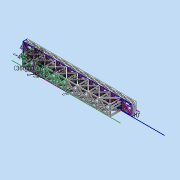
# Autodesk Inventor part: hashi1shado
Saved by Autodesk Inventor 2022 (Build 260153000, 153)
## iProperties
Created: 2024-05-14
Part Number: hashi1shado
Material: 一般
Document SubType Name: Modeling
Designer: ktamu
Density: 1 g/cm^3
Appearance: 既定
Mass: 212.611 g
Surface Area: 1968.28 cm^2
Volume: 212.611 cm^3
Author: ktamu
Autodesk Inventor part; units mm, degrees
(part 1 of 2)
ref_plane "YZ Plane" through (0, 0, 0) normal (1, 0, 0) x (0, 1, 0)
ref_plane "XZ Plane" through (0, 0, 0) normal (0, 1, 0) x (-1, 0, 0)
ref_plane "XY Plane" through (0, 0, 0) normal (0, 0, 1) x (1, 0, 0)
sketch "スケッチ2" plane through (0, 0, 0) normal (1, 0, 0) x (0, 1, 0)
  line L0 (25, 10) -> (-25, 10)
  line L1 (-25, 10) -> (-25, -10)
  line L2 (-25, -10) -> (25, -10)
  line L3 (25, -10) -> (25, 10)
  line L4 (25, 10) -> (-25, -10) construction
  line L5 (-25, 10) -> (25, -10) construction
  point P0 (0, 0)
  dimension "d4" = 50
  dimension "d5" = 20
  constraints: 12 end point, 2 midpoint, 2 parallel, 1 horizontal, 1 perpendicular
  measures "d4" distance of L2.end L1.end
  measures "d5" distance of L1.end L0.end
extrude "押し出し2" add sketch "スケッチ2" along normal mid plane 500
sketch "スケッチ3" plane through (-250, -25, 10) normal (0, 0, 1) x (1, 0, 0)
  circle A0 centre (250, 25) radius 5
  dimension "d8" = 10
  constraints: 1 centre point, 1 coincident
  measures "d8" diameter of A0
extrude "押し出し3" add sketch "スケッチ3" along normal blind 2
sketch "SCfront" plane through (-250, -25, 10) normal (0, -1, 0) x (1, 0, 0)
  line L0 (0, -20) -> (500, -20) projected
  line L1 (500, 0) -> (500, -20) projected
  line L2 (500, 0) -> (0, 0) projected
  line L3 (0, -20) -> (0, 0) projected
  line L4 (0, 0) -> (500, 0)
  line L5 (500, 0) -> (500, -20)
  line L6 (500, -20) -> (0, -20)
  line L7 (0, -20) -> (0, 0)
  line L8 (0, 0) -> (500, -20) construction
  line L9 (500, 0) -> (0, -20) construction
  line L10 (0, 0) -> (500, 0) projected
  line L11 (0, -20) -> (500, -20) projected
  line L12 (0, 0) -> (50, 0)
  line L13 (50, 0) -> (50, -20)
  line L14 (50, -20) -> (0, -20)
  line L15 (0, -20) -> (0, 0)
  line L16 (100, 0) -> (100, -20)
  line L17 (150, 0) -> (150, -20)
  line L18 (200, 0) -> (200, -20)
  line L19 (250, 0) -> (250, -20)
  line L20 (450, 0) -> (450, -20)
  line L21 (400, 0) -> (400, -20)
  line L22 (350, 0) -> (350, -20)
  line L23 (300, 0) -> (300, -20)
  line L24 (0, 0) -> (0, -20) projected
  line L25 (0, 0) -> (50, -20)
  line L26 (0, -20) -> (50, 0) construction
  line L27 (50, 0) -> (100, -20)
  line L28 (100, 0) -> (50, -20)
  line L29 (52, -4) -> (98, -4)
  line L30 (98, -4) -> (98, -16)
  line L31 (98, -16) -> (52, -16)
  line L32 (52, -16) -> (52, -4)
  line L33 (75, -10) -> (98, -16) construction
  line L34 (98, -4) -> (52, -16) construction
  line L35 (102, -4) -> (148, -4)
  line L36 (102, -16) -> (102, -4)
  line L37 (148, -16) -> (102, -16)
  line L38 (148, -4) -> (148, -16)
  line L39 (152, -4) -> (198, -4)
  line L40 (152, -16) -> (152, -4)
  line L41 (198, -16) -> (152, -16)
  line L42 (198, -4) -> (198, -16)
  line L43 (202, -4) -> (248, -4)
  line L44 (202, -16) -> (202, -4)
  line L45 (248, -16) -> (202, -16)
  line L46 (248, -4) -> (248, -16)
  line L47 (252, -4) -> (298, -4)
  line L48 (252, -16) -> (252, -4)
  line L49 (298, -16) -> (252, -16)
  line L50 (298, -4) -> (298, -16)
  line L51 (302, -4) -> (348, -4)
  line L52 (302, -16) -> (302, -4)
  line L53 (348, -16) -> (302, -16)
  line L54 (348, -4) -> (348, -16)
  line L55 (352, -4) -> (398, -4)
  line L56 (352, -16) -> (352, -4)
  line L57 (398, -16) -> (352, -16)
  line L58 (398, -4) -> (398, -16)
  line L59 (402, -4) -> (448, -4)
  line L60 (402, -16) -> (402, -4)
  line L61 (448, -16) -> (402, -16)
  line L62 (448, -4) -> (448, -16)
  line L63 (48, -4) -> (48, -16)
  line L64 (48, -4) -> (4, -4)
  line L65 (4, -4) -> (4, -16.3421)
  line L66 (4, -16.3421) -> (48, -16.3421)
  line L67 (48, -16.3421) -> (48, -4)
  line L68 (452, -4) -> (452, -16)
  line L69 (452, -4) -> (496, -4)
  line L70 (496, -4) -> (496, -16.3421)
  line L71 (496, -16.3421) -> (452, -16.3421)
  line L72 (11.4052, -4) -> (48, -14.2649)
  line L73 (4, -6.0772) -> (40.5948, -16.3421)
  line L74 (488.5948, -4) -> (452, -14.2649)
  line L75 (496, -6.0772) -> (459.4052, -16.3421)
  line L76 (52, -4) -> (75, -10)
  line L77 (52, -6.0669) -> (90.0768, -16)
  line L78 (52.5048, -2.0648) -> (52.6652, -2.1066)
  line L79 (59.9232, -4) -> (98, -13.9331)
  line L80 (109.9232, -4) -> (148, -13.9331)
  line L81 (102, -6.0669) -> (140.0768, -16)
  line L82 (159.9232, -4) -> (198, -13.9331)
  line L83 (152, -6.0669) -> (190.0768, -16)
  line L84 (209.9232, -4) -> (248, -13.9331)
  line L85 (202, -6.0669) -> (240.0768, -16)
  line L86 (448, -6.0669) -> (409.9232, -16)
  line L87 (440.0768, -4) -> (402, -13.9331)
  line L88 (390.0768, -4) -> (352, -13.9331)
  line L89 (398, -6.0669) -> (359.9232, -16)
  line L90 (340.0768, -4) -> (302, -13.9331)
  line L91 (348, -6.0669) -> (309.9232, -16)
  line L92 (290.0768, -4) -> (252, -13.9331)
  line L93 (298, -6.0669) -> (259.9232, -16)
  line L94 (0, -10) -> (496, -10) construction
  line L95 (0, -10) -> (496, -10) construction
  line L96 (11.4052, -16) -> (48, -5.7351)
  line L97 (4, -13.9228) -> (39.375, -4)
  line L98 (488.5948, -16) -> (452, -5.7351)
  line L99 (496, -13.9228) -> (459.4052, -3.6579)
  line L100 (52, -13.9331) -> (90.0768, -4)
  line L101 (59.9232, -16) -> (98, -6.0669)
  line L102 (109.9232, -16) -> (148, -6.0669)
  line L103 (102, -13.9331) -> (140.0768, -4)
  line L104 (159.9232, -16) -> (198, -6.0669)
  line L105 (152, -13.9331) -> (190.0768, -4)
  line L106 (209.9232, -16) -> (248, -6.0669)
  line L107 (202, -13.9331) -> (240.0768, -4)
  line L108 (448, -13.9331) -> (409.9232, -4)
  line L109 (440.0768, -16) -> (402, -6.0669)
  line L110 (398, -13.9331) -> (359.9232, -4)
  line L111 (390.0768, -16) -> (352, -6.0669)
  line L112 (348, -13.9331) -> (309.9232, -4)
  line L113 (340.0768, -16) -> (302, -6.0669)
  line L114 (298, -13.9331) -> (259.9232, -4)
  line L115 (290.0768, -16) -> (252, -6.0669)
  line L116 (25.3901, -12.0772) -> (10.1855, -16.3421)
  line L117 (474.6099, -12.0772) -> (489.8145, -16.3421)
  line L118 (50.8793, -20) -> (54.8793, -20)
  line L119 (54.8793, -20) -> (54.8793, -36)
  line L120 (54.8793, -36) -> (50.8793, -36)
  line L121 (50.8793, -36) -> (50.8793, -20)
  line L122 (500, -20) -> (0, -20)
  line L123 (0, -36) -> (500, -36)
  line L124 (445.1207, -20) -> (445.1207, -36)
  line L125 (449.1207, -36) -> (449.1207, -20)
  line L126 (50, 0) -> (100, 0)
  line L127 (100, 0) -> (100, 50)
  line L128 (100, 50) -> (50, 50)
  line L129 (50, 50) -> (50, 0)
  line L130 (50, 50) -> (100, 0)
  line L131 (50, 0) -> (100, 50)
  line L132 (50, 0) -> (100, 0)
  line L133 (54.8284, 48) -> (95.1716, 48)
  line L134 (95.1716, 48) -> (75, 27.8284)
  line L135 (75, 27.8284) -> (54.8284, 48)
  line L136 (52, 4.8284) -> (52, 45.1716)
  line L137 (72.1716, 25) -> (52, 4.8284)
  line L138 (52, 45.1716) -> (72.1716, 25)
  line L139 (95.1716, 2) -> (54.8284, 2)
  line L140 (75, 22.1716) -> (95.1716, 2)
  line L141 (54.8284, 2) -> (75, 22.1716)
  line L142 (98, 45.1716) -> (98, 4.8284)
  line L143 (77.8284, 25) -> (98, 45.1716)
  line L144 (98, 4.8284) -> (77.8284, 25)
  line L145 (55.944, 3.1156) -> (52.8284, 0)
  line L146 (93.8909, 3.2807) -> (97.1716, 0)
  line L147 (150, 50) -> (100, 50)
  line L148 (104.8284, 48) -> (145.1716, 48)
  line L149 (145.1716, 48) -> (125, 27.8284)
  line L150 (125, 27.8284) -> (104.8284, 48)
  line L151 (102, 4.8284) -> (102, 45.1716)
  line L152 (102, 45.1716) -> (122.1716, 25)
  line L153 (122.1716, 25) -> (102, 4.8284)
  line L154 (127.8284, 25) -> (148, 45.1716)
  line L155 (148, 45.1716) -> (148, 4.8284)
  line L156 (148, 4.8284) -> (127.8284, 25)
  line L157 (104.8284, 2) -> (125, 22.1716)
  line L158 (125, 22.1716) -> (145.1716, 2)
  line L159 (143.8909, 3.2807) -> (147.1716, 0)
  line L160 (50, 0) -> (550, 0)
  line L161 (105.944, 3.1156) -> (102.8284, 0)
  line L162 (200, 50) -> (150, 50)
  line L163 (154.8284, 48) -> (195.1716, 48)
  line L164 (195.1716, 48) -> (175, 27.8284)
  line L165 (175, 27.8284) -> (154.8284, 48)
  line L166 (152, 4.8284) -> (152, 45.1716)
  line L167 (152, 45.1716) -> (172.1716, 25)
  line L168 (172.1716, 25) -> (152, 4.8284)
  line L169 (177.8284, 25) -> (198, 45.1716)
  line L170 (198, 45.1716) -> (198, 4.8284)
  line L171 (198, 4.8284) -> (177.8284, 25)
  line L172 (154.8284, 2) -> (175, 22.1716)
  line L173 (175, 22.1716) -> (195.1716, 2)
  line L174 (193.8909, 3.2807) -> (197.1716, 0)
  line L175 (100, 0) -> (600, 0)
  line L176 (155.944, 3.1156) -> (152.8284, 0)
  line L177 (250, 50) -> (200, 50)
  line L178 (204.8284, 48) -> (245.1716, 48)
  line L179 (245.1716, 48) -> (225, 27.8284)
  line L180 (225, 27.8284) -> (204.8284, 48)
  line L181 (202, 4.8284) -> (202, 45.1716)
  line L182 (202, 45.1716) -> (222.1716, 25)
  line L183 (222.1716, 25) -> (202, 4.8284)
  line L184 (227.8284, 25) -> (248, 45.1716)
  line L185 (248, 45.1716) -> (248, 4.8284)
  line L186 (248, 4.8284) -> (227.8284, 25)
  line L187 (204.8284, 2) -> (225, 22.1716)
  line L188 (225, 22.1716) -> (245.1716, 2)
  line L189 (243.8909, 3.2807) -> (247.1716, 0)
  line L190 (150, 0) -> (650, 0)
  line L191 (205.944, 3.1156) -> (202.8284, 0)
  line L192 (250, 50) -> (250, 0)
  line L193 (250, 50) -> (250, 52)
  line L194 (250, 52) -> (50, 52)
  line L195 (50, 52) -> (50, 50)
  point P0 (250, -10)
  point P1 (440.0768, -4)
  point P2 (390.0768, -4)
  point P3 (340.0768, -4)
  point P4 (290.0768, -4)
  point P5 (209.9232, -4)
  point P6 (159.9232, -4)
  point P7 (109.9232, -4)
  point P8 (60.1439, -4.0576)
  point P9 (60, -4)
  point P10 (90, -16)
  point P11 (89.8561, -15.9424)
  point P12 (48, -14.2649)
  point P13 (40.5948, -3.6579)
  point P14 (482.0151, -10)
  point P15 (474.6099, -7.9228)
  point P16 (460.625, -4)
  point P17 (467.2046, -10)
  point P18 (432.9232, -10)
  point P19 (425, -12.0669)
  point P20 (425, -7.9331)
  point P21 (417.0768, -10)
  point P22 (382.9232, -10)
  point P23 (375, -12.0669)
  point P24 (375, -7.9331)
  point P25 (367.0768, -10)
  point P26 (332.9232, -10)
  point P27 (325, -12.0669)
  point P28 (325, -7.9331)
  point P29 (317.0768, -10)
  point P30 (282.9232, -10)
  point P31 (275, -12.0669)
  point P32 (275, -7.9331)
  point P33 (267.0768, -10)
  point P34 (232.9232, -10)
  point P35 (225, -7.9331)
  point P36 (225, -12.0669)
  point P37 (217.0768, -10)
  point P38 (182.9232, -10)
  point P39 (175, -7.9331)
  point P40 (175, -12.0669)
  point P41 (167.0768, -10)
  point P42 (132.9232, -10)
  point P43 (125, -7.9331)
  point P44 (125, -12.0669)
  point P45 (117.0768, -10)
  point P46 (67.0768, -10)
  point P47 (59.9232, -16)
  point P48 (75, -12.0669)
  point P49 (75, -7.9331)
  point P50 (82.9232, -10)
  point P51 (25.3901, -7.9228)
  point P52 (32.7954, -10)
  point P53 (48, -5.7351)
  point P54 (11.4052, -16)
  point P55 (17.9849, -10)
  point P56 (4, -13.9228)
  point P57 (54.8793, -20)
  point P58 (75, 25)
  point P59 (202.8284, 0)
  point P60 (152.8284, 0)
  point P61 (102.8284, 0)
  point P62 (54.8284, 2)
  point P63 (52.8284, 0)
  dimension "d12" = 50
  dimension "d15" = 50
  dimension "d20" = 46
  dimension "d21" = 12
  dimension "d24" = 50
  dimension "d29" = 4
  dimension "d30" = 4
  dimension "d33" = 4
  dimension "d37" = 2
  dimension "d40" = 50
  dimension "d96" = 0
  dimension "d97" = 10
  dimension "d116" = 4
  dimension "d125" = 50
  dimension "d126" = 50
  dimension "d132" = 2
  dimension "d133" = 2
  dimension "d134" = 2
  dimension "d137" = 360
  dimension "d141" = 50
  dimension "d146" = 2
  constraints: 378 end point, 79 symmetric about line, 41 point on line, 18 parallel, 12 horizontal, 7 midpoint, 6 perpendicular, 3 collinear, 1 vertical, 215 other
  measures "d12" distance of L13.end L14.end
  measures "d15" distance of L12.end L16.start
  measures "d20" distance of L30.end L31.end
  measures "d21" distance of L29.end L30.end
  measures "d24" distance of L29.start L35.start
  measures "d29" distance between parallel lines of L32 L63
  measures "d30" distance between parallel lines of L65 L3
  measures "d33" distance between parallel lines of L12 L64
  measures "d37" distance between parallel lines of L76 L77
  measures "d40" distance of L79.start L80.start
  measures "d96" distance between parallel lines of L94 L95
  measures "d97" distance between parallel lines of L0 L95
  measures "d116" distance of L119.end L120.end
  measures "d125" distance of L128.end L127.end
  measures "d126" distance of L127.end L126.end
  measures "d132" distance between parallel lines of L130 L135
  measures "d133" distance between parallel lines of L128 L133
  measures "d134" distance between parallel lines of L131 L134
  measures "d141" distance of L127.end L147.start
  measures "d146" distance of L193.end L193.start
extrude "押し出し4" cut sketch "SCfront" against normal through all contours L31 L101 L28 | L28 L101 L77 L27 L31 | L29 L28 L100 L79 L27 | L66 L116 L96 L73 | L101 L31 L32 L100 L77 L28 | L28 L77 L101 | L64 L97 L72 | L29 L100 L28 | L96 L116 L66 L65 L97 L73 | L96 L63 L72 | L72 L97 L64 L63 L96 | L97 L65 L73 | L100 L28 L79 | L100 L29 L30 L101 L79 L28 | L100 L32 L77 | L101 L30 L79 | L35 L103 L80 | L81 L103 L36 | L35 L38 L102 L80 L103 | L103 L81 L102 L37 L36 | L102 L38 L80 | L81 L37 L102 | L39 L105 L82 | L83 L105 L40 | L39 L42 L104 L82 L105 | L105 L83 L104 L41 L40 | L104 L42 L82 | L83 L41 L104 | L43 L107 L84 | L85 L107 L44 | L43 L46 L106 L84 L107 | L107 L85 L106 L45 L44 | L106 L46 L84 | L85 L45 L106 | L47 L114 L92 L115 L48 | L47 L92 L114 | L115 L92 L48 | L114 L50 L49 L115 L93 | L93 L50 L114 | L115 L49 L93 | L51 L112 L90 L113 L52 | L51 L90 L112 | L113 L90 L52 | L112 L54 L53 L113 L91 | L91 L54 L112 | L113 L53 L91 | L55 L110 L88 L111 L56 | L55 L88 L110 | L111 L88 L56 | L110 L58 L57 L111 L89 | L89 L58 L110 | L111 L57 L89 | L59 L108 L87 L109 L60 | L59 L87 L108 | L109 L87 L60 | L108 L62 L61 L109 L86 | L86 L62 L108 | L109 L61 L86 | L69 L99 L74 L98 L68 | L98 L74 L68 | L69 L74 L99 | L98 L117 L71 L75 | L75 L99 L70 L71 L117 L98 | L75 L70 L99
sketch "SCLeft" plane through (-250, 0, 0) normal (-1, 0, 0) x (0, 0, 1)
  line L0 (10, 25) -> (10, -25) projected
  line L1 (-10, 25) -> (10, 25)
  line L2 (10, 25) -> (10, -25)
  line L3 (10, -25) -> (-10, -25)
  line L4 (-10, -25) -> (-10, 25)
  line L5 (-10, 25) -> (10, -25) construction
  line L6 (10, 25) -> (-10, -25) construction
  line L7 (-6, 21) -> (6, 21)
  line L8 (6, 21) -> (6, -21)
  line L9 (6, -21) -> (-6, -21)
  line L10 (-6, -21) -> (-6, 21)
  line L11 (-6, 21) -> (-1.04, 3.6401) construction
  line L12 (6, 21) -> (-6, -21) construction
  line L13 (7.4154, 0) -> (4.3427, 0)
  line L14 (2.08, 0) -> (6, -13.7199)
  line L15 (-3.92, 21) -> (0, 7.2801)
  line L16 (-6, 21) -> (-1.04, 3.6401)
  line L17 (1.04, -3.6401) -> (6, -21)
  line L18 (-6, 13.7199) -> (-2.08, 0)
  line L19 (0, -7.2801) -> (3.92, -21)
  line L20 (0, 7.2801) -> (3.92, 21)
  line L21 (-6, -13.7199) -> (-2.08, 0)
  line L22 (-3.92, -21) -> (0, -7.2801)
  line L23 (2.08, 0) -> (6, 13.7199)
  point P0 (0, 0)
  dimension "d47" = 12
  dimension "d48" = 42
  constraints: 46 end point, 8 parallel, 5 point on line, 4 symmetric about line, 3 horizontal, 3 midpoint, 2 perpendicular
  measures "d47" distance of L8.end L9.end
  measures "d48" distance of L7.end L8.end
extrude "押し出し5left" cut sketch "SCLeft" against normal through all contours L7 L15 L20 L8 L23 L14 L9 L19 L22 L10 L21 L18 | L7 L20 L15 | L18 L21 L10 | L8 L14 L23 | L22 L19 L9
extrude "押し出し6" add sketch "SCLeft" against normal blind 4 contours L7 L15 L20 L8 L23 L14 L9 L19 L22 L10 L21 L18
mirror "ミラー1" about plane through (0, 0, 0) normal (1, 0, 0) of "押し出し6"
sketch "SCtop" plane through (-250, -25, 10) normal (0, 0, 1) x (1, 0, 0)
  circle A0 centre (250, 25) radius 5 projected
  line L0 (500, 0) -> (0, 0) projected
  line L1 (500, 50) -> (500, 0) projected
  line L2 (0, 50) -> (500, 50) projected
  line L3 (0, 0) -> (0, 50) projected
  circle A1 centre (250, 25) radius 5 projected
  line L4 (0, 0) -> (0, 50) projected
  line L5 (0, 50) -> (500, 0) construction
  line L6 (0, 0) -> (500, 0) projected
  line L7 (500, 50) -> (0, 0) construction
  line L8 (0, 50) -> (500, 50)
  line L9 (500, 50) -> (500, 0)
  line L10 (500, 0) -> (0, 0)
  line L11 (0, 0) -> (0, 50)
  line L12 (0, 50) -> (500, 0) construction
  line L13 (500, 50) -> (0, 0) construction
  line L14 (0, 50) -> (500, 50) projected
  line L15 (0, 50) -> (50, 50)
  line L16 (50, 50) -> (50, 0)
  line L17 (50, 0) -> (0, 0)
  line L18 (0, 0) -> (0, 50)
  line L19 (100, 50) -> (100, 0)
  line L20 (150, 50) -> (150, 0)
  line L21 (200, 50) -> (200, 0)
  line L22 (250, 50) -> (250, 0)
  line L23 (300, 50) -> (300, 0)
  line L24 (350, 50) -> (350, 0)
  line L25 (400, 50) -> (400, 0)
  line L26 (450, 50) -> (450, 0)
  line L27 (50, 50) -> (100, 0)
  line L28 (0, 50) -> (50, 0)
  line L29 (50, 50) -> (0, 0)
  line L30 (98, 4) -> (60.1439, 4) projected
  line L31 (52, 46) -> (98, 46)
  line L32 (98, 46) -> (98, 4)
  line L33 (98, 4) -> (52, 4)
  line L34 (52, 4) -> (52, 46)
  line L35 (4, 46) -> (48, 46)
  line L36 (48, 46) -> (48, 4)
  line L37 (48, 4) -> (4, 4)
  line L38 (4, 4) -> (4, 46)
  line L39 (6.8284, 46) -> (48.0258, 4.8026)
  line L40 (4, 43.1716) -> (43.1716, 4)
  line L41 (25, 25) -> (25, 18.6219)
  line L42 (98, 0) -> (98, 4) projected
  line L43 (53.4759, 44.6524) -> (98, 4)
  line L44 (52, 43.2918) -> (95.0338, 4)
  line L45 (54.9662, 46) -> (98, 6.7082)
  line L46 (98, 43.2918) -> (54.9662, 4)
  line L47 (92.2747, 40.7725) -> (53.4759, 5.3476)
  line L48 (95.0338, 46) -> (52, 6.7082)
  line L49 (50.1449, 5.0145) -> (50, 4.8822)
  line L50 (73.5843, 23.5843) -> (90.9091, 40.9091)
  line L51 (92.2747, 40.7725) -> (73.5169, 23.6459) construction
  line L52 (53.4759, 5.3476) -> (52, 4) construction
  line L53 (52, 46) -> (53.4759, 44.6524) construction
  line L54 (73.5169, 26.3541) -> (98, 4) construction
  line L55 (48, 46) -> (4, 4)
  line L56 (45.1034, 46) -> (4, 6.7649)
  line L57 (48, 43.2351) -> (6.8966, 4)
  line L58 (104.9662, 46) -> (148, 6.7082)
  line L59 (145.0338, 46) -> (102, 6.7082)
  line L60 (148, 43.2918) -> (104.9662, 4)
  line L61 (102, 43.2918) -> (145.0338, 4)
  line L62 (148, 46) -> (148, 4)
  line L63 (102, 46) -> (148, 46)
  line L64 (102, 4) -> (102, 46)
  line L65 (148, 4) -> (102, 4)
  line L66 (154.9662, 46) -> (198, 6.7082)
  line L67 (195.0338, 46) -> (152, 6.7082)
  line L68 (198, 43.2918) -> (154.9662, 4)
  line L69 (152, 43.2918) -> (195.0338, 4)
  line L70 (198, 46) -> (198, 4)
  line L71 (152, 46) -> (198, 46)
  line L72 (152, 4) -> (152, 46)
  line L73 (198, 4) -> (152, 4)
  line L74 (204.9662, 46) -> (248, 6.7082)
  line L75 (245.0338, 46) -> (202, 6.7082)
  line L76 (248, 43.2918) -> (204.9662, 4)
  line L77 (202, 43.2918) -> (245.0338, 4)
  line L78 (248, 46) -> (248, 4)
  line L79 (202, 46) -> (248, 46)
  line L80 (202, 4) -> (202, 46)
  line L81 (248, 4) -> (202, 4)
  line L82 (254.9662, 46) -> (298, 6.7082)
  line L83 (295.0338, 46) -> (252, 6.7082)
  line L84 (298, 43.2918) -> (254.9662, 4)
  line L85 (252, 43.2918) -> (295.0338, 4)
  line L86 (298, 46) -> (298, 4)
  line L87 (252, 46) -> (298, 46)
  line L88 (252, 4) -> (252, 46)
  line L89 (298, 4) -> (252, 4)
  line L90 (304.9662, 46) -> (348, 6.7082)
  line L91 (345.0338, 46) -> (302, 6.7082)
  line L92 (348, 43.2918) -> (304.9662, 4)
  line L93 (302, 43.2918) -> (345.0338, 4)
  line L94 (348, 46) -> (348, 4)
  line L95 (302, 46) -> (348, 46)
  line L96 (302, 4) -> (302, 46)
  line L97 (348, 4) -> (302, 4)
  line L98 (354.9662, 46) -> (398, 6.7082)
  line L99 (395.0338, 46) -> (352, 6.7082)
  line L100 (398, 43.2918) -> (354.9662, 4)
  line L101 (352, 43.2918) -> (395.0338, 4)
  line L102 (398, 46) -> (398, 4)
  line L103 (352, 46) -> (398, 46)
  line L104 (352, 4) -> (352, 46)
  line L105 (398, 4) -> (352, 4)
  line L106 (404.9662, 46) -> (448, 6.7082)
  line L107 (445.0338, 46) -> (402, 6.7082)
  line L108 (448, 43.2918) -> (404.9662, 4)
  line L109 (402, 43.2918) -> (445.0338, 4)
  line L110 (448, 46) -> (448, 4)
  line L111 (402, 46) -> (448, 46)
  line L112 (402, 4) -> (402, 46)
  line L113 (448, 4) -> (402, 4)
  line L114 (496, 46) -> (452, 46)
  line L115 (452, 46) -> (452, 4)
  line L116 (452, 4) -> (496, 4)
  line L117 (496, 4) -> (496, 46)
  line L118 (493.1716, 46) -> (451.9742, 4.8026)
  line L119 (496, 43.1716) -> (456.8284, 4)
  line L120 (454.8966, 46) -> (496, 6.7649)
  line L121 (452, 43.2351) -> (493.1034, 4)
  point P0 (75, 25)
  point P1 (123.5169, 26.3541)
  point P2 (123.5843, 23.5843)
  point P3 (123.5169, 23.6459)
  point P4 (173.5169, 26.3541)
  point P5 (173.5843, 23.5843)
  point P6 (173.5169, 23.6459)
  point P7 (223.5169, 26.3541)
  point P8 (223.5843, 23.5843)
  point P9 (223.5169, 23.6459)
  point P10 (273.5169, 26.3541)
  point P11 (273.5843, 23.5843)
  point P12 (273.5169, 23.6459)
  point P13 (323.5169, 26.3541)
  point P14 (323.5843, 23.5843)
  point P15 (323.5169, 23.6459)
  point P16 (373.5169, 26.3541)
  point P17 (373.5843, 23.5843)
  point P18 (373.5169, 23.6459)
  point P19 (423.5169, 26.3541)
  point P20 (423.5843, 23.5843)
  point P21 (423.5169, 23.6459)
  point P22 (474.5441, 21.7157)
  point P23 (477.3733, 24.5449)
  point P24 (474.4791, 27.3075)
  point P25 (452, 4.8284)
  point P26 (471.6499, 24.4784)
  point P27 (427.9662, 25)
  point P28 (425, 22.2918)
  point P29 (425, 27.7082)
  point P30 (375, 22.2918)
  point P31 (375, 27.7082)
  point P32 (422.0338, 25)
  point P33 (377.9662, 25)
  point P34 (372.0338, 25)
  point P35 (327.9662, 25)
  point P36 (325, 22.2918)
  point P37 (325, 27.7082)
  point P38 (322.0338, 25)
  point P39 (275, 22.2918)
  point P40 (277.9662, 25)
  point P41 (275, 27.7082)
  point P42 (252, 20.4174)
  point P43 (272.0338, 25)
  point P44 (252, 29.5826)
  point P45 (225, 22.2918)
  point P46 (248, 29.5826)
  point P47 (227.9662, 25)
  point P48 (248, 20.4174)
  point P49 (225, 27.7082)
  point P50 (222.0338, 25)
  point P51 (175, 22.2918)
  point P52 (177.9662, 25)
  point P53 (175, 27.7082)
  point P54 (172.0338, 25)
  point P55 (125, 22.2918)
  point P56 (127.9662, 25)
  point P57 (125, 27.7082)
  point P58 (122.0338, 25)
  point P59 (77.9662, 25)
  point P60 (75, 22.2918)
  point P61 (75, 27.7082)
  point P62 (72.0338, 25)
  point P63 (25.4559, 21.7157)
  point P64 (28.3501, 24.4784)
  point P65 (48, 4.8284)
  point P66 (22.6267, 24.5449)
  point P67 (25.5209, 27.3075)
  dimension "d55" = 50
  dimension "d56" = 50
  dimension "d59" = 50
  dimension "d64" = 46
  dimension "d65" = 42
  dimension "d66" = 44
  dimension "d67" = 42
  dimension "d68" = 4
  dimension "d69" = 4
  dimension "d76" = 2
  dimension "d77" = 2
  dimension "d80" = 50
  constraints: 226 end point, 97 point on line, 20 midpoint, 17 parallel, 12 symmetric about line, 6 horizontal, 5 perpendicular, 1 vertical, 185 other
  measures "d55" distance of L16.end L17.end
  measures "d56" distance of L15.end L16.end
  measures "d59" distance of L15.end L19.start
  measures "d64" distance of L30.start L33.end
  measures "d65" distance of L31.end L30.start
  measures "d66" distance of L36.end L37.end
  measures "d67" distance of L35.end L36.end
  measures "d68" distance between parallel lines of L2 L35
  measures "d69" distance between parallel lines of L34 L36
  measures "d76" distance between parallel lines of L55 L56
  measures "d77" distance between parallel lines of L55 L57
  measures "d80" distance of L45.start L58.start
extrude "押し出し7" cut sketch "SCtop" against normal through all contours A0 L88 L85 L83 | A0 L78 L74 L76 | L82 L87 L83 | L85 L89 L84 | L84 L86 L82 | L74 L79 L75 | L77 L81 L76 | L75 L80 L77 | L31 L48 L45 | L56 L39 L35 | L30 L33 L46 L44 | L45 L46 L32 | L40 L56 L38 | L44 L48 L34 | L36 L39 L57 | L37 L57 L40 | L63 L59 L58 | L60 L62 L58 | L59 L64 L61 | L61 L65 L60 | L71 L67 L66 | L68 L70 L66 | L67 L72 L69 | L69 L73 L68 | L95 L91 L90 | L92 L94 L90 | L91 L96 L93 | L93 L97 L92 | L103 L99 L98 | L100 L102 L98 | L99 L104 L101 | L101 L105 L100 | L111 L107 L106 | L108 L110 L106 | L107 L112 L109 | L109 L113 L108 | L118 L120 L114 | L117 L120 L119 | L118 L115 L121 | L121 L116 L119
sketch "スケッチ7" plane through (0, 0, 12) normal (0, 0, 1) x (1, 0, 0)
  line L0 (-2, 21) -> (-2, -21) projected
  line L1 (2, -18.2918) -> (2, -4.5826) projected
  line L2 (2, -21) -> (2, 21) projected
  circle A0 centre (0, 0) radius 5 projected
  arc A1 (-2, -4.5826) -> (2, -4.5826) centre (0, 0) ccw projected
  line L3 (-2, -4.5826) -> (-2, 4.5826)
  line L4 (2, -4.5826) -> (2, 4.5826)
  circle A2 centre (0, 0) radius 1
  point P0 (-2, -4.5826)
  dimension "d89" = 2
  constraints: 4 end point, 2 point on circle, 2 point on line, 1 centre point, 1 coincident
  measures "d89" diameter of A2
extrude "押し出し8" cut sketch "スケッチ7" against normal through all contours L0 A0 | A0 L2
extrude "押し出し9" cut sketch "スケッチ7" against normal blind 2 contours A0 L2 L0
extrude "押し出し10" cut sketch "スケッチ7" against normal blind 1 contours A2
extrude "押し出し11" cut sketch "スケッチ7" against normal blind 2 contours A2
extrude "押し出し12" add sketch "SCfront" against normal blind 4 contours L101 L31 L32 L100 L77 L28 | L28 L77 L101 | L96 L116 L66 L65 L97 L73 | L72 L97 L64 L63 L96 | L100 L28 L79 | L100 L29 L30 L101 L79 L28 | L35 L38 L102 L80 L103 | L103 L81 L102 L37 L36 | L39 L42 L104 L82 L105 | L105 L83 L104 L41 L40 | L43 L46 L106 L84 L107 | L107 L85 L106 L45 L44 | L47 L114 L92 L115 L48 | L114 L50 L49 L115 L93 | L51 L112 L90 L113 L52 | L112 L54 L53 L113 L91 | L55 L110 L88 L111 L56 | L110 L58 L57 L111 L89 | L59 L108 L87 L109 L60 | L108 L62 L61 L109 L86 | L69 L99 L74 L98 L68 | L98 L117 L71 L75 | L75 L99 L70 L71 L117 L98
extrude "押し出し13" cut sketch "SCfront" against normal blind 88.5 contours L98 L117 L71 L75
mirror "ミラー2" about plane through (0, 0, 0) normal (0, 1, 0) of "押し出し12"
extrude "押し出し14" cut sketch "SCfront" against normal blind 84 contours L98 L117 L71 L75
sketch "スケッチ8" plane through (-250, -25, 10) normal (0, 0, 1) x (1, 0, 0)
  line L0 (252, 6.7082) -> (252, 43.2918) projected
  line L1 (252, 43.2918) -> (272.0338, 25) projected
  line L2 (272.0338, 25) -> (252, 6.7082) projected
  line L3 (248, 43.2918) -> (248, 6.7082) projected
  line L4 (248, 6.7082) -> (227.9662, 25) projected
  line L5 (227.9662, 25) -> (248, 43.2918) projected
  line L6 (48, 43.2351) -> (48, 4.8284) projected
  line L7 (48, 4.8284) -> (28.3501, 24.4784) projected
  line L8 (28.3501, 24.4784) -> (48, 43.2351) projected
  line L9 (75, 22.2918) -> (95.0338, 4) projected
  line L10 (95.0338, 4) -> (54.9662, 4) projected
  line L11 (54.9662, 4) -> (75, 22.2918) projected
  line L12 (148, 6.7082) -> (127.9662, 25) projected
  line L13 (127.9662, 25) -> (148, 43.2918) projected
  line L14 (148, 43.2918) -> (148, 6.7082) projected
  line L15 (198, 6.7082) -> (177.9662, 25) projected
  line L16 (177.9662, 25) -> (198, 43.2918) projected
  line L17 (198, 43.2918) -> (198, 6.7082) projected
  line L18 (298, 6.7082) -> (277.9662, 25) projected
  line L19 (277.9662, 25) -> (298, 43.2918) projected
  line L20 (298, 43.2918) -> (298, 6.7082) projected
  line L21 (304.9662, 4) -> (325, 22.2918) projected
  line L22 (325, 22.2918) -> (345.0338, 4) projected
  line L23 (345.0338, 4) -> (304.9662, 4) projected
  line L24 (402, 43.2918) -> (422.0338, 25) projected
  line L25 (422.0338, 25) -> (402, 6.7082) projected
  line L26 (402, 6.7082) -> (402, 43.2918) projected
  line L27 (404.9662, 4) -> (425, 22.2918) projected
  line L28 (425, 22.2918) -> (445.0338, 4) projected
  line L29 (445.0338, 4) -> (404.9662, 4) projected
  line L30 (496, 6.7649) -> (477.3733, 24.5449) projected
  line L31 (477.3733, 24.5449) -> (496, 43.1716) projected
  line L32 (496, 43.1716) -> (496, 6.7649) projected
  line L33 (493.1716, 46) -> (474.4791, 27.3075) projected
  line L34 (474.4791, 27.3075) -> (454.8966, 46) projected
  line L35 (454.8966, 46) -> (493.1716, 46) projected
  line L36 (445.0338, 46) -> (425, 27.7082) projected
  line L37 (425, 27.7082) -> (404.9662, 46) projected
  line L38 (404.9662, 46) -> (445.0338, 46) projected
  line L39 (398, 6.7082) -> (377.9662, 25) projected
  line L40 (377.9662, 25) -> (398, 43.2918) projected
  line L41 (398, 43.2918) -> (398, 6.7082) projected
  line L42 (345.0338, 46) -> (325, 27.7082) projected
  line L43 (325, 27.7082) -> (304.9662, 46) projected
  line L44 (304.9662, 46) -> (345.0338, 46) projected
  line L45 (295.0338, 46) -> (275, 27.7082) projected
  line L46 (275, 27.7082) -> (254.9662, 46) projected
  line L47 (254.9662, 46) -> (295.0338, 46) projected
  line L48 (245.0338, 46) -> (225, 27.7082) projected
  line L49 (225, 27.7082) -> (204.9662, 46) projected
  line L50 (204.9662, 46) -> (245.0338, 46) projected
  line L51 (195.0338, 46) -> (175, 27.7082) projected
  line L52 (175, 27.7082) -> (154.9662, 46) projected
  line L53 (154.9662, 46) -> (195.0338, 46) projected
  line L54 (145.0338, 46) -> (125, 27.7082) projected
  line L55 (125, 27.7082) -> (104.9662, 46) projected
  line L56 (104.9662, 46) -> (145.0338, 46) projected
  line L57 (75, 27.7082) -> (54.9662, 46) projected
  line L58 (54.9662, 46) -> (95.0338, 46) projected
  line L59 (95.0338, 46) -> (75, 27.7082) projected
  line L60 (4, 6.7649) -> (4, 43.1716) projected
  line L61 (4, 43.1716) -> (22.6267, 24.5449) projected
  line L62 (22.6267, 24.5449) -> (4, 6.7649) projected
  line L63 (25.4559, 21.7157) -> (43.1716, 4) projected
  line L64 (43.1716, 4) -> (6.8966, 4) projected
  line L65 (6.8966, 4) -> (25.4559, 21.7157) projected
  line L66 (98, 43.2918) -> (98, 6.7082) projected
  line L67 (98, 6.7082) -> (77.9662, 25) projected
  line L68 (77.9662, 25) -> (98, 43.2918) projected
  line L69 (104.9662, 4) -> (125, 22.2918) projected
  line L70 (125, 22.2918) -> (145.0338, 4) projected
  line L71 (145.0338, 4) -> (104.9662, 4) projected
  line L72 (154.9662, 4) -> (175, 22.2918) projected
  line L73 (175, 22.2918) -> (195.0338, 4) projected
  line L74 (195.0338, 4) -> (154.9662, 4) projected
  line L75 (204.9662, 4) -> (225, 22.2918) projected
  line L76 (225, 22.2918) -> (245.0338, 4) projected
  line L77 (245.0338, 4) -> (204.9662, 4) projected
  line L78 (254.9662, 4) -> (275, 22.2918) projected
  line L79 (275, 22.2918) -> (295.0338, 4) projected
  line L80 (295.0338, 4) -> (254.9662, 4) projected
  line L81 (348, 6.7082) -> (327.9662, 25) projected
  line L82 (327.9662, 25) -> (348, 43.2918) projected
  line L83 (348, 43.2918) -> (348, 6.7082) projected
  line L84 (395.0338, 46) -> (375, 27.7082) projected
  line L85 (375, 27.7082) -> (354.9662, 46) projected
  line L86 (354.9662, 46) -> (395.0338, 46) projected
  line L87 (448, 6.7082) -> (427.9662, 25) projected
  line L88 (427.9662, 25) -> (448, 43.2918) projected
  line L89 (448, 43.2918) -> (448, 6.7082) projected
  line L90 (456.8284, 4) -> (474.5441, 21.7157) projected
  line L91 (474.5441, 21.7157) -> (493.1034, 4) projected
  line L92 (493.1034, 4) -> (456.8284, 4) projected
  line L93 (452, 43.2351) -> (471.6499, 24.4784) projected
  line L94 (471.6499, 24.4784) -> (452, 4.8284) projected
  line L95 (452, 4.8284) -> (452, 43.2351) projected
  line L96 (354.9662, 4) -> (375, 22.2918) projected
  line L97 (375, 22.2918) -> (395.0338, 4) projected
  line L98 (395.0338, 4) -> (354.9662, 4) projected
  line L99 (352, 43.2918) -> (372.0338, 25) projected
  line L100 (372.0338, 25) -> (352, 6.7082) projected
  line L101 (352, 6.7082) -> (352, 43.2918) projected
  line L102 (302, 43.2918) -> (322.0338, 25) projected
  line L103 (322.0338, 25) -> (302, 6.7082) projected
  line L104 (302, 6.7082) -> (302, 43.2918) projected
  line L105 (202, 43.2918) -> (222.0338, 25) projected
  line L106 (222.0338, 25) -> (202, 6.7082) projected
  line L107 (202, 6.7082) -> (202, 43.2918) projected
  line L108 (152, 43.2918) -> (172.0338, 25) projected
  line L109 (172.0338, 25) -> (152, 6.7082) projected
  line L110 (152, 6.7082) -> (152, 43.2918) projected
  line L111 (102, 43.2918) -> (122.0338, 25) projected
  line L112 (122.0338, 25) -> (102, 6.7082) projected
  line L113 (102, 6.7082) -> (102, 43.2918) projected
  line L114 (52, 6.7082) -> (52, 43.2918) projected
  line L115 (52, 43.2918) -> (72.0338, 25) projected
  line L116 (72.0338, 25) -> (52, 6.7082) projected
  line L117 (25.5209, 27.3075) -> (6.8284, 46) projected
  line L118 (6.8284, 46) -> (45.1034, 46) projected
  line L119 (45.1034, 46) -> (25.5209, 27.3075) projected
  line L120 (500, 0) -> (0, 0) projected
  line L121 (500, 50) -> (500, 0) projected
  line L122 (0, 50) -> (500, 50) projected
  line L123 (0, 0) -> (0, 50) projected
  line L124 (252, 6.7082) -> (252, 43.2918) projected
  line L125 (252, 43.2918) -> (272.0338, 25) projected
  line L126 (272.0338, 25) -> (252, 6.7082) projected
  line L127 (248, 43.2918) -> (248, 6.7082) projected
  line L128 (248, 6.7082) -> (227.9662, 25) projected
  line L129 (227.9662, 25) -> (248, 43.2918) projected
  line L130 (48, 43.2351) -> (48, 4.8284) projected
  line L131 (48, 4.8284) -> (28.3501, 24.4784) projected
  line L132 (28.3501, 24.4784) -> (48, 43.2351) projected
  line L133 (75, 22.2918) -> (95.0338, 4) projected
  line L134 (95.0338, 4) -> (54.9662, 4) projected
  line L135 (54.9662, 4) -> (75, 22.2918) projected
  line L136 (148, 6.7082) -> (127.9662, 25) projected
  line L137 (127.9662, 25) -> (148, 43.2918) projected
  line L138 (148, 43.2918) -> (148, 6.7082) projected
  line L139 (198, 6.7082) -> (177.9662, 25) projected
  line L140 (177.9662, 25) -> (198, 43.2918) projected
  line L141 (198, 43.2918) -> (198, 6.7082) projected
  line L142 (298, 6.7082) -> (277.9662, 25) projected
  line L143 (277.9662, 25) -> (298, 43.2918) projected
  line L144 (298, 43.2918) -> (298, 6.7082) projected
  line L145 (304.9662, 4) -> (325, 22.2918) projected
  line L146 (325, 22.2918) -> (345.0338, 4) projected
  line L147 (345.0338, 4) -> (304.9662, 4) projected
  line L148 (402, 43.2918) -> (422.0338, 25) projected
  line L149 (422.0338, 25) -> (402, 6.7082) projected
  line L150 (402, 6.7082) -> (402, 43.2918) projected
  line L151 (404.9662, 4) -> (425, 22.2918) projected
  line L152 (425, 22.2918) -> (445.0338, 4) projected
  line L153 (445.0338, 4) -> (404.9662, 4) projected
  line L154 (496, 6.7649) -> (477.3733, 24.5449) projected
  line L155 (477.3733, 24.5449) -> (496, 43.1716) projected
  line L156 (496, 43.1716) -> (496, 6.7649) projected
  line L157 (493.1716, 46) -> (474.4791, 27.3075) projected
  line L158 (474.4791, 27.3075) -> (454.8966, 46) projected
  line L159 (454.8966, 46) -> (493.1716, 46) projected
  line L160 (445.0338, 46) -> (425, 27.7082) projected
  line L161 (425, 27.7082) -> (404.9662, 46) projected
  line L162 (404.9662, 46) -> (445.0338, 46) projected
  line L163 (398, 6.7082) -> (377.9662, 25) projected
  line L164 (377.9662, 25) -> (398, 43.2918) projected
  line L165 (398, 43.2918) -> (398, 6.7082) projected
  line L166 (345.0338, 46) -> (325, 27.7082) projected
  line L167 (325, 27.7082) -> (304.9662, 46) projected
  line L168 (304.9662, 46) -> (345.0338, 46) projected
  line L169 (295.0338, 46) -> (275, 27.7082) projected
  line L170 (275, 27.7082) -> (254.9662, 46) projected
  line L171 (254.9662, 46) -> (295.0338, 46) projected
  line L172 (245.0338, 46) -> (225, 27.7082) projected
  line L173 (225, 27.7082) -> (204.9662, 46) projected
  line L174 (204.9662, 46) -> (245.0338, 46) projected
  line L175 (195.0338, 46) -> (175, 27.7082) projected
  line L176 (175, 27.7082) -> (154.9662, 46) projected
  line L177 (154.9662, 46) -> (195.0338, 46) projected
  line L178 (145.0338, 46) -> (125, 27.7082) projected
  line L179 (125, 27.7082) -> (104.9662, 46) projected
  line L180 (104.9662, 46) -> (145.0338, 46) projected
  line L181 (75, 27.7082) -> (54.9662, 46) projected
  line L182 (54.9662, 46) -> (95.0338, 46) projected
  line L183 (95.0338, 46) -> (75, 27.7082) projected
  line L184 (4, 6.7649) -> (4, 43.1716) projected
  line L185 (4, 43.1716) -> (22.6267, 24.5449) projected
  line L186 (22.6267, 24.5449) -> (4, 6.7649) projected
  line L187 (25.4559, 21.7157) -> (43.1716, 4) projected
  line L188 (43.1716, 4) -> (6.8966, 4) projected
  line L189 (6.8966, 4) -> (25.4559, 21.7157) projected
  line L190 (98, 43.2918) -> (98, 6.7082) projected
  line L191 (98, 6.7082) -> (77.9662, 25) projected
  line L192 (77.9662, 25) -> (98, 43.2918) projected
  line L193 (104.9662, 4) -> (125, 22.2918) projected
  line L194 (125, 22.2918) -> (145.0338, 4) projected
  line L195 (145.0338, 4) -> (104.9662, 4) projected
  line L196 (154.9662, 4) -> (175, 22.2918) projected
  line L197 (175, 22.2918) -> (195.0338, 4) projected
  line L198 (195.0338, 4) -> (154.9662, 4) projected
  line L199 (204.9662, 4) -> (225, 22.2918) projected
  line L200 (225, 22.2918) -> (245.0338, 4) projected
  line L201 (245.0338, 4) -> (204.9662, 4) projected
  line L202 (254.9662, 4) -> (275, 22.2918) projected
  line L203 (275, 22.2918) -> (295.0338, 4) projected
  line L204 (295.0338, 4) -> (254.9662, 4) projected
  line L205 (348, 6.7082) -> (327.9662, 25) projected
  line L206 (327.9662, 25) -> (348, 43.2918) projected
  line L207 (348, 43.2918) -> (348, 6.7082) projected
  line L208 (395.0338, 46) -> (375, 27.7082) projected
  line L209 (375, 27.7082) -> (354.9662, 46) projected
  line L210 (354.9662, 46) -> (395.0338, 46) projected
  line L211 (448, 6.7082) -> (427.9662, 25) projected
  line L212 (427.9662, 25) -> (448, 43.2918) projected
  line L213 (448, 43.2918) -> (448, 6.7082) projected
  line L214 (456.8284, 4) -> (474.5441, 21.7157) projected
  line L215 (474.5441, 21.7157) -> (493.1034, 4) projected
  line L216 (493.1034, 4) -> (456.8284, 4) projected
  line L217 (452, 43.2351) -> (471.6499, 24.4784) projected
  line L218 (471.6499, 24.4784) -> (452, 4.8284) projected
  line L219 (452, 4.8284) -> (452, 43.2351) projected
  line L220 (354.9662, 4) -> (375, 22.2918) projected
  line L221 (375, 22.2918) -> (395.0338, 4) projected
  line L222 (395.0338, 4) -> (354.9662, 4) projected
  line L223 (352, 43.2918) -> (372.0338, 25) projected
  line L224 (372.0338, 25) -> (352, 6.7082) projected
  line L225 (352, 6.7082) -> (352, 43.2918) projected
  line L226 (302, 43.2918) -> (322.0338, 25) projected
  line L227 (322.0338, 25) -> (302, 6.7082) projected
  line L228 (302, 6.7082) -> (302, 43.2918) projected
  line L229 (202, 43.2918) -> (222.0338, 25) projected
  line L230 (222.0338, 25) -> (202, 6.7082) projected
  line L231 (202, 6.7082) -> (202, 43.2918) projected
  line L232 (152, 43.2918) -> (172.0338, 25) projected
  line L233 (172.0338, 25) -> (152, 6.7082) projected
  line L234 (152, 6.7082) -> (152, 43.2918) projected
  line L235 (102, 43.2918) -> (122.0338, 25) projected
  line L236 (122.0338, 25) -> (102, 6.7082) projected
  line L237 (102, 6.7082) -> (102, 43.2918) projected
  line L238 (52, 6.7082) -> (52, 43.2918) projected
  line L239 (52, 43.2918) -> (72.0338, 25) projected
  line L240 (72.0338, 25) -> (52, 6.7082) projected
  line L241 (25.5209, 27.3075) -> (6.8284, 46) projected
  line L242 (6.8284, 46) -> (45.1034, 46) projected
  line L243 (45.1034, 46) -> (25.5209, 27.3075) projected
  line L244 (500, 0) -> (0, 0) projected
  line L245 (500, 50) -> (500, 0) projected
  line L246 (0, 50) -> (500, 50) projected
  line L247 (0, 0) -> (0, 50) projected
  line L248 (48, 46) -> (48, 50) projected
  line L249 (0, 0) -> (500, 0) projected
  line L250 (48, 50) -> (250, 50)
  line L251 (250, 50) -> (250, 0)
  line L252 (250, 0) -> (48, 0)
  line L253 (48, 0) -> (48, 50)
  point P0 (250, 25)
  constraints: 8 end point, 2 parallel, 1 horizontal, 1 midpoint, 1 perpendicular
extrude "押し出し20" add sketch "スケッチ8" along normal blind 52 contours L3 L4 L5 | L253 L248 L122 L251 L120 L6 | L9 L10 L11 | L12 L13 L14 | L15 L16 L17 | L48 L49 L50 | L51 L52 L53 | L54 L55 L56 | L57 L58 L59 | L66 L67 L68 | L69 L70 L71 | L72 L73 L74 | L75 L76 L77 | L105 L106 L107 | L108 L109 L110 | L111 L112 L113 | L114 L115 L116
sketch "スケッチ9" plane through (-250, -25, 62) normal (0, 0, 1) x (1, 0, 0)
  line L0 (250, 25) -> (48, 25)
  line L1 (48, 4.8284) -> (48, 43.2351) projected
  line L2 (250, 27) -> (48, 27)
  line L3 (250, 23) -> (48, 23)
  line L4 (48, 50) -> (48, 0) projected
  line L5 (48, 0) -> (250, 0) projected
  line L6 (250, 0) -> (250, 50) projected
  line L7 (250, 50) -> (48, 50) projected
  line L8 (50, 0) -> (100, 0)
  line L9 (100, 0) -> (100, 50)
  line L10 (100, 50) -> (50, 50)
  line L11 (50, 50) -> (50, 0)
  line L12 (50, 50) -> (96, 4)
  line L13 (50, 0) -> (100, 50)
  line L14 (50, 0) -> (100, 0)
  line L15 (54.8284, 48) -> (95.1716, 48)
  line L16 (95.1716, 48) -> (75, 27.8284)
  line L17 (75, 27.8284) -> (54.8284, 48)
  line L18 (52, 4.8284) -> (52, 45.1716)
  line L19 (72.1716, 25) -> (52, 4.8284)
  line L20 (52, 45.1716) -> (72.1716, 25)
  line L21 (95.1716, 2) -> (54.8284, 2)
  line L22 (75, 22.1716) -> (95.1716, 2)
  line L23 (54.8284, 2) -> (75, 22.1716)
  line L24 (98, 45.1716) -> (98, 4.8284)
  line L25 (77.8284, 25) -> (98, 45.1716)
  line L26 (98, 4.8284) -> (77.8284, 25)
  line L27 (55.944, 3.1156) -> (52.8284, 0)
  line L28 (150, 50) -> (100, 50)
  line L29 (143.1716, 46) -> (125, 27.8284)
  line L30 (125, 27.8284) -> (106.8284, 46)
  line L31 (102, 4.8284) -> (102, 45.1716)
  line L32 (102, 45.1716) -> (122.1716, 25)
  line L33 (122.1716, 25) -> (102, 4.8284)
  line L34 (127.8284, 25) -> (148, 45.1716)
  line L35 (148, 45.1716) -> (148, 4.8284)
  line L36 (148, 4.8284) -> (127.8284, 25)
  line L37 (106.8284, 4) -> (125, 22.1716)
  line L38 (125, 22.1716) -> (145.1716, 2)
  line L39 (143.8909, 3.2807) -> (145.1716, 2)
  line L40 (105.944, 3.1156) -> (104.8284, 2)
  line L41 (200, 50) -> (150, 50)
  line L42 (193.1716, 46) -> (175, 27.8284)
  line L43 (175, 27.8284) -> (156.8284, 46)
  line L44 (152, 4.8284) -> (152, 45.1716)
  line L45 (152, 45.1716) -> (172.1716, 25)
  line L46 (172.1716, 25) -> (152, 4.8284)
  line L47 (177.8284, 25) -> (198, 45.1716)
  line L48 (198, 45.1716) -> (198, 4.8284)
  line L49 (198, 4.8284) -> (177.8284, 25)
  line L50 (154.8284, 2) -> (175, 22.1716)
  line L51 (175, 22.1716) -> (195.1716, 2)
  line L52 (193.8909, 3.2807) -> (195.1716, 2)
  line L53 (250, 50) -> (200, 50)
  line L54 (243.1716, 46) -> (225, 27.8284)
  line L55 (225, 27.8284) -> (206.8284, 46)
  line L56 (202, 4.8284) -> (202, 45.1716)
  line L57 (202, 45.1716) -> (222.1716, 25)
  line L58 (222.1716, 25) -> (202, 4.8284)
  line L59 (227.8284, 25) -> (248, 45.1716)
  line L60 (248, 45.1716) -> (248, 4.8284)
  line L61 (248, 4.8284) -> (227.8284, 25)
  line L62 (204.8284, 2) -> (225, 22.1716)
  line L63 (225, 22.1716) -> (245.1716, 2)
  line L64 (243.8909, 3.2807) -> (245.1716, 2)
  line L65 (250, 50) -> (250, 0)
  line L66 (250, 50) -> (250, 52)
  line L67 (250, 52) -> (50, 52)
  line L68 (50, 52) -> (50, 50)
  line L69 (48, 4) -> (32.7954, 4) projected
  line L70 (48, 4) -> (250, 4)
  line L71 (48, 46) -> (250, 46)
  point P0 (150, 0)
  point P1 (200, 0)
  point P2 (75, 25)
  point P3 (150, 0)
  point P4 (98, 23)
  point P5 (79.8284, 23)
  point P6 (56.8284, 4)
  point P7 (93.1716, 4)
  point P8 (70.1716, 23)
  point P9 (52, 23)
  point P10 (52, 27)
  point P11 (70.1716, 27)
  point P12 (98, 27)
  point P13 (79.8284, 27)
  point P14 (93.1716, 46)
  point P15 (56.8284, 46)
  point P16 (143.1716, 4)
  point P17 (148, 23)
  point P18 (129.8284, 23)
  point P19 (120.1716, 23)
  point P20 (102, 23)
  point P21 (120.1716, 27)
  point P22 (102, 27)
  point P23 (148, 27)
  point P24 (129.8284, 27)
  point P25 (156.8284, 4)
  point P26 (193.1716, 4)
  point P27 (170.1716, 23)
  point P28 (152, 23)
  point P29 (152, 27)
  point P30 (170.1716, 27)
  point P31 (198, 23)
  point P32 (179.8284, 23)
  point P33 (179.8284, 27)
  point P34 (198, 27)
  point P35 (220.1716, 23)
  point P36 (202, 23)
  point P37 (220.1716, 27)
  point P38 (202, 27)
  point P39 (248, 27)
  point P40 (229.8284, 27)
  point P41 (229.8284, 23)
  point P42 (248, 23)
  point P43 (206.8284, 4)
  point P44 (243.1716, 4)
  dimension "d149" = 2
  dimension "d150" = 2
  dimension "d153" = 50
  dimension "d154" = 50
  dimension "d155" = 50
  dimension "d156" = 2
  dimension "d157" = 2
  dimension "d158" = 2
  dimension "d159" = 360
  dimension "d160" = 50
  dimension "d161" = 2
  dimension "d172" = 2
  constraints: 132 end point, 23 point on line, 7 parallel, 3 horizontal, 2 perpendicular, 2 symmetric about line, 1 midpoint, 25 other
  measures "d149" distance between parallel lines of L0 L2
  measures "d150" distance between parallel lines of L0 L3
  measures "d153" distance of L8.start point (100, 0)
  measures "d154" distance of L10.end L9.end
  measures "d155" distance of L9.end L9.start
  measures "d156" distance between parallel lines of L12 L17
  measures "d157" distance between parallel lines of L10 L15
  measures "d158" distance between parallel lines of L13 L16
  measures "d160" distance of L9.end L28.start
  measures "d161" distance of L66.end L66.start
  measures "d172" distance between parallel lines of L5 L21
sketch "スケッチ10" plane through (0, -25, 10) normal (1, 0, 0) x (0, 0, -1)
  line L0 (0, 50) -> (0, 46) projected
  line L1 (0, 50) -> (-52, 50) projected
  line L2 (-52, 0) -> (-52, 50) projected
  line L3 (0, 0) -> (-52, 0) projected
  line L4 (0, 4) -> (-48, 4) projected
  line L5 (-48, 4) -> (-48, 46) projected
  line L6 (-48, 46) -> (0, 46) projected
  line L7 (0, 4) -> (0, 0) projected
  point P0 (10, 25)
sketch "スケッチ11" plane through (0, -25, 10) normal (1, 0, 0) x (0, 0, -1)
  line L0 (-48, 4) -> (0, 4)
  line L1 (0, 4) -> (0, 46)
  line L2 (0, 46) -> (-48, 46)
  line L3 (-48, 46) -> (-48, 4)
  line L4 (0, 50) -> (-52, 50) projected
  line L5 (-52, 0) -> (-52, 50) projected
  line L6 (0, 0) -> (-52, 0) projected
  line L7 (0, 50) -> (0, 0) projected
  point P0 (10, 25)
  dimension "d162" = 4
  dimension "d163" = 4
  dimension "d164" = 4
  dimension "d165" = 0
  constraints: 8 end point, 2 parallel, 1 horizontal, 1 perpendicular
  measures "d162" distance between parallel lines of L4 L2
  measures "d163" distance between parallel lines of L5 L3
  measures "d164" distance between parallel lines of L6 L0
  measures "d165" distance between parallel lines of L7 L1
extrude "押し出し21" cut sketch "スケッチ11" against normal through all contours L3 L2 L1 L0
sketch "スケッチ12" plane through (-202, -25, 10) normal (-1, 0, 0) x (0, 0, 1)
  line L0 (48, 46) -> (0, 46) projected
  line L1 (0, 4) -> (-4, 4) projected
  line L2 (48, 46) -> (0, 4)
  line L3 (0, 4) -> (48, 4)
  line L4 (48, 4) -> (0, 46)
  line L5 (0, 46) -> (24, 46)
  line L6 (24, 46) -> (24, 4)
  line L7 (0, 25) -> (48, 25)
  line L8 (0, 23) -> (48, 23)
  line L9 (0, 27) -> (48, 27)
  line L10 (48, 4) -> (0, 4) projected
  line L11 (0, 0) -> (0, 4) projected
  line L12 (0, 0) -> (52, 0) projected
  line L13 (52, 50) -> (52, 0) projected
  line L14 (0, 50) -> (52, 50) projected
  line L15 (0, 46) -> (0, 50) projected
  line L16 (0, 46) -> (48, 46) projected
  line L17 (48, 46) -> (48, 4) projected
  line L18 (-13.92, 46) -> (-6.08, 46) projected
  line L19 (-6.08, 46) -> (-10, 32.2801) projected
  line L20 (-10, 32.2801) -> (-13.92, 46) projected
  line L21 (-16, 38.7199) -> (-12.08, 25) projected
  line L22 (-12.08, 25) -> (-16, 11.2801) projected
  line L23 (-16, 11.2801) -> (-16, 38.7199) projected
  line L24 (-13.92, 4) -> (-10, 17.7199) projected
  line L25 (-10, 17.7199) -> (-6.08, 4) projected
  line L26 (-6.08, 4) -> (-13.92, 4) projected
  line L27 (-4, 11.2801) -> (-7.92, 25) projected
  line L28 (-7.92, 25) -> (-4, 38.7199) projected
  line L29 (-4, 38.7199) -> (-4, 11.2801) projected
  line L30 (-20, 0) -> (0, 0) projected
  line L31 (0, 0) -> (0, 50) projected
  line L32 (0, 50) -> (-20, 50) projected
  line L33 (-20, 50) -> (-20, 0) projected
  line L34 (0, 27) -> (0, 23)
  point P0 (-10, 25)
  dimension "d168" = 2
  dimension "d169" = 2
  constraints: 18 end point, 3 parallel, 2 collinear, 2 midpoint, 2 perpendicular, 2 point on line, 1 horizontal
  measures "d168" distance between parallel lines of L7 L8
  measures "d169" distance between parallel lines of L7 L9
extrude "押し出し22" cut sketch "SCfront" against normal through all contours L145 L139 L146 L2 | L141 L140 L139 | L161 L157 L158 L159 L2 | L176 L172 L173 L174 L2 | L191 L187 L188 L189 L2 | L133 L134 L135 | L136 L138 L137 | L142 L144 L143 | L148 L149 L150 | L151 L152 L153 | L154 L155 L156 | L163 L164 L165 | L166 L167 L168 | L169 L170 L171 | L178 L179 L180 | L181 L182 L183 | L184 L185 L186
extrude "押し出し23" cut sketch "スケッチ9" against normal blind 10 contours L59 L60 L2 | L3 L60 L61 | L2 L56 L57 | L58 L56 L3 | L2 L47 L48 | L48 L49 L3 | L70 L62 L63 | L54 L55 L71 | L2 L44 L45 | L46 L44 L3 | L70 L50 L51 | L42 L43 L71 | L2 L34 L35 | L35 L36 L3 | L37 L38 L70 | L3 L33 L31 | L24 L26 L3 | L70 L23 L22 | L29 L30 L71 | L2 L31 L32 | L16 L17 L71 | L3 L19 L18 | L2 L25 L24 | L18 L20 L2
sketch "スケッチ13" plane through (-250, -25, 62) normal (0, 0, 1) x (1, 0, 0)
  line L0 (229.8284, 23) -> (248, 23) projected
  line L1 (248, 23) -> (248, 4.8284) projected
  line L2 (248, 4.8284) -> (229.8284, 23) projected
  line L3 (198, 45.1716) -> (198, 27) projected
  line L4 (198, 27) -> (179.8284, 27) projected
  line L5 (179.8284, 27) -> (198, 45.1716) projected
  line L6 (152, 4.8284) -> (152, 23) projected
  line L7 (152, 23) -> (170.1716, 23) projected
  line L8 (170.1716, 23) -> (152, 4.8284) projected
  line L9 (120.1716, 27) -> (102, 27) projected
  line L10 (102, 27) -> (102, 45.1716) projected
  line L11 (102, 45.1716) -> (120.1716, 27) projected
  line L12 (93.1716, 46) -> (75, 27.8284) projected
  line L13 (75, 27.8284) -> (56.8284, 46) projected
  line L14 (56.8284, 46) -> (93.1716, 46) projected
  line L15 (56.8284, 4) -> (75, 22.1716) projected
  line L16 (75, 22.1716) -> (93.1716, 4) projected
  line L17 (93.1716, 4) -> (56.8284, 4) projected
  line L18 (52, 4.8284) -> (52, 23) projected
  line L19 (52, 23) -> (70.1716, 23) projected
  line L20 (70.1716, 23) -> (52, 4.8284) projected
  line L21 (106.8284, 4) -> (125, 22.1716) projected
  line L22 (125, 22.1716) -> (143.1716, 4) projected
  line L23 (143.1716, 4) -> (106.8284, 4) projected
  line L24 (148, 27) -> (129.8284, 27) projected
  line L25 (129.8284, 27) -> (148, 45.1716) projected
  line L26 (148, 45.1716) -> (148, 27) projected
  line L27 (152, 45.1716) -> (170.1716, 27) projected
  line L28 (170.1716, 27) -> (152, 27) projected
  line L29 (152, 27) -> (152, 45.1716) projected
  line L30 (202, 4.8284) -> (202, 23) projected
  line L31 (202, 23) -> (220.1716, 23) projected
  line L32 (220.1716, 23) -> (202, 4.8284) projected
  line L33 (206.8284, 4) -> (225, 22.1716) projected
  line L34 (225, 22.1716) -> (243.1716, 4) projected
  line L35 (243.1716, 4) -> (206.8284, 4) projected
  line L36 (248, 27) -> (229.8284, 27) projected
  line L37 (229.8284, 27) -> (248, 45.1716) projected
  line L38 (248, 45.1716) -> (248, 27) projected
  line L39 (198, 4.8284) -> (179.8284, 23) projected
  line L40 (179.8284, 23) -> (198, 23) projected
  line L41 (198, 23) -> (198, 4.8284) projected
  line L42 (156.8284, 4) -> (175, 22.1716) projected
  line L43 (175, 22.1716) -> (193.1716, 4) projected
  line L44 (193.1716, 4) -> (156.8284, 4) projected
  line L45 (102, 4.8284) -> (102, 23) projected
  line L46 (102, 23) -> (120.1716, 23) projected
  line L47 (120.1716, 23) -> (102, 4.8284) projected
  line L48 (98, 27) -> (79.8284, 27) projected
  line L49 (79.8284, 27) -> (98, 45.1716) projected
  line L50 (98, 45.1716) -> (98, 27) projected
  line L51 (98, 4.8284) -> (79.8284, 23) projected
  line L52 (79.8284, 23) -> (98, 23) projected
  line L53 (98, 23) -> (98, 4.8284) projected
  line L54 (52, 45.1716) -> (70.1716, 27) projected
  line L55 (70.1716, 27) -> (52, 27) projected
  line L56 (52, 27) -> (52, 45.1716) projected
  line L57 (148, 4.8284) -> (129.8284, 23) projected
  line L58 (129.8284, 23) -> (148, 23) projected
  line L59 (148, 23) -> (148, 4.8284) projected
  line L60 (143.1716, 46) -> (125, 27.8284) projected
  line L61 (125, 27.8284) -> (106.8284, 46) projected
  line L62 (106.8284, 46) -> (143.1716, 46) projected
  line L63 (193.1716, 46) -> (175, 27.8284) projected
  line L64 (175, 27.8284) -> (156.8284, 46) projected
  line L65 (156.8284, 46) -> (193.1716, 46) projected
  line L66 (220.1716, 27) -> (202, 27) projected
  line L67 (202, 27) -> (202, 45.1716) projected
  line L68 (202, 45.1716) -> (220.1716, 27) projected
  line L69 (243.1716, 46) -> (225, 27.8284) projected
  line L70 (225, 27.8284) -> (206.8284, 46) projected
  line L71 (206.8284, 46) -> (243.1716, 46) projected
  line L72 (48, 50) -> (48, 0) projected
  line L73 (48, 0) -> (250, 0) projected
  line L74 (250, 0) -> (250, 50) projected
  line L75 (250, 50) -> (48, 50) projected
  line L76 (0, 0) -> (500, 0) projected
  line L77 (98, 50) -> (102, 50)
  line L78 (102, 50) -> (102, 0)
  line L79 (102, 0) -> (98, 0)
  line L80 (98, 0) -> (98, 50)
  point P0 (250, 25)
  constraints: 8 end point, 2 parallel, 2 point on line, 1 horizontal, 1 perpendicular
pattern_linear "矩形状パターン2" count 2 spacing 200 along (1, 0, 0) of "押し出し22", "押し出し23", "押し出し20", "押し出し21"